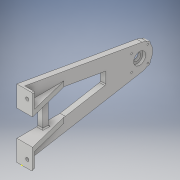
# Autodesk Inventor part: halter_seite
Saved by Autodesk Inventor 2017 (Build 210142000, 142)
## iProperties
Part Number: halter_seite
Material: Generisch
Document SubType Name: Modeling
Designer: Fabio
Density: 1 g/cm^3
Appearance: Vorgabe
Author: Fabio
Autodesk Inventor part; units mm, degrees
ref_plane "YZ Plane" through (0, 0, 0) normal (1, 0, 0) x (0, 1, 0)
ref_plane "XZ Plane" through (0, 0, 0) normal (0, 1, 0) x (-1, 0, 0)
ref_plane "XY Plane" through (0, 0, 0) normal (0, 0, 1) x (1, 0, 0)
sketch "Skizze1" plane through (0, 0, 0) normal (1, 0, 0) x (0, 1, 0)
  arc A0 (250, 65.0592) -> (229.3412, 89.6794) centre (225, 65.0592) ccw
  line L0 (225, 65.0592) -> (229.3412, 89.6794) construction
  line L1 (225, 65.0592) -> (250, 65.0592) construction
  line L2 (229.3412, 89.6794) -> (0, 130.1185)
  line L3 (0, 130.1185) -> (0, 90.1185)
  arc A1 (229.3412, 40.439) -> (250, 65.0592) centre (225, 65.0592) ccw
  line L4 (229.3412, 40.439) -> (0, 0)
  line L5 (0, 0) -> (92.864, 0) construction
  line L6 (0, 0) -> (0, 40)
  line L7 (160, 76.5205) -> (160, 53.598)
  line L8 (40, 90.1185) -> (40, 40)
  line L9 (50, 40) -> (50, 90.1185)
  line L10 (82.882, 90.1185) -> (160, 76.5205)
  line L11 (82.882, 40) -> (160, 53.598)
  line L12 (0, 40) -> (40, 40)
  line L13 (50, 40) -> (82.882, 40)
  line L14 (0, 90.1185) -> (40, 90.1185)
  line L15 (50, 90.1185) -> (82.882, 90.1185)
  dimension "d21" = 80
  dimension "d24" = 25
  dimension "d68" = 250
  dimension "d73" = 80
  dimension "d88" = 130.1185
  dimension "d91" = 10
  dimension "d92" = 25
  dimension "d93" = 25
  dimension "d94" = 40
  dimension "d127" = 110
  dimension "d160" = 40
  dimension "d161" = 40
  dimension "d162" = 80
  dimension "d163" = 32.882
  dimension "d164" = 32.882
  constraints: 32 end point, 5 horizontal, 4 point on circle, 4 vertical, 2 centre point, 2 symmetric about line, 1 coincident, 1 parallel, 1 other
  measures "d21" angle of L1 L0
  measures "d24" radius of A0
  measures "d68" distance from line of L1.end L3
  measures "d73" angle of L3 L2
  measures "d88" distance of point (0, 0) L2.end
  measures "d91" distance between parallel lines of L8 L9
  measures "d92" distance between parallel lines of L2 L10
  measures "d93" distance between parallel lines of L4 L11
  measures "d94" distance from line of L8 L3.end
  measures "d127" distance between parallel lines of L9 L7
  measures "d160" distance of L2.end L3.end
  measures "d161" distance of L4.end L6.end
  measures "d162" angle of L4 L6
  measures "d163" distance of L9.end L10.start
  measures "d164" distance of L9.start L11.start
extrude "Extrusion2" add sketch "Skizze1" along normal blind 10
sketch "Skizze7" plane through (10, 0, 0) normal (1, 0, 0) x (0, 0, -1)
  arc A0 (-40.439, 229.3412) -> (-89.6794, 229.3412) centre (-65.0592, 225) ccw projected
  point P0 (0, 0)
  constraints: 1 coincident
hole "Bohrung6" at (10, 225, 65.0592) direction (-1, 0, 0) diameter 14 end through all
fillet "Rundung1" radius 2 5 edges at (5, 160, 76.5205) (5, 40, 90.1185) (5, 50, 40) (5, 160, 53.598) (5, 40, 40)
sketch "Skizze13" plane through (0, 0, 0) normal (-1, 0, 0) x (0, 0, 1)
  line L0 (80.5592, 240.5) -> (80.5592, 209.5)
  line L1 (80.5592, 209.5) -> (49.5592, 209.5)
  line L2 (49.5592, 209.5) -> (49.5592, 240.5)
  line L3 (49.5592, 240.5) -> (80.5592, 240.5)
  line L4 (80.5592, 240.5) -> (49.5592, 209.5) construction
  line L5 (80.5592, 209.5) -> (49.5592, 240.5) construction
  line L6 (80.5592, 240.5) -> (111.5592, 240.5) construction
  point P0 (0, 0)
  point P1 (65.0592, 225)
  dimension "d145" = 31
  dimension "d146" = 90
  dimension "d147" = 31
  constraints: 14 end point, 4 coincident, 2 midpoint, 2 parallel, 2 perpendicular, 1 horizontal
  measures "d145" distance of L0.start L0.end
  measures "d146" angle of L0 L6
  measures "d147" distance of L0.end L1.end
hole "Bohrung10" at (0, 209.5, 80.5592) at (0, 240.5, 80.5592) at (0, 240.5, 49.5592) at (0, 209.5, 49.5592) direction (1, 0, 0) diameter 3 end through all counterbore diameter 5 counterbore depth 5
sketch "Skizze14" plane through (10, 0, 0) normal (1, 0, 0) x (0, 0, -1)
  line L0 (-90.1185, 0) -> (-90.1185, 38) projected
  line L1 (-90.1185, 0) -> (-100.1185, 0)
  line L2 (-100.1185, 0) -> (-100.1185, 80)
  line L3 (-100.1185, 80) -> (-90.1185, 80)
  line L4 (-90.1185, 80) -> (-90.1185, 0)
  line L5 (-40, 0) -> (0, 0) projected
  line L6 (-40, 0) -> (-30, 0)
  line L7 (-30, 0) -> (-30, 80)
  line L8 (-30, 80) -> (-40, 80)
  line L9 (-40, 80) -> (-40, 0)
  dimension "d165" = 10
  dimension "d166" = 80
  dimension "d167" = 10
  dimension "d168" = 80
  constraints: 16 end point, 4 parallel, 2 horizontal, 2 perpendicular
  measures "d165" distance of L2.end L3.end
  measures "d166" distance of L1.end L2.end
  measures "d167" distance of L8.end L7.end
  measures "d168" distance of L7.end L6.end
sketch "Skizze15" plane through (10, 0, 0) normal (1, 0, 0) x (0, 0, -1)
  circle A0 centre (-65.0592, 225) radius 7 projected
  circle A1 centre (-65.0592, 225) radius 11.5
  point P0 (0, 0)
  dimension "d157" = 23
  constraints: 1 centre point, 1 coincident
  measures "d157" diameter of A1
extrude "Extrusion4" cut sketch "Skizze15" against normal blind 5
sketch "Skizze16" plane through (10, 0, 0) normal (1, 0, 0) x (0, 0, -1)
  point P0 (0, 0)
sketch "Skizze17" plane through (10, 0, 0) normal (1, 0, 0) x (0, 0, -1)
  point P0 (0, 0)
extrude "Extrusion5" add sketch "Skizze14" along normal blind 20
sketch "Skizze18" plane through (10, 0, 100.1185) normal (0, 0, 1) x (1, 0, 0)
  line L0 (0, 0) -> (0, 80) projected
  line L1 (0, 0) -> (20, 0) projected
  line L2 (20, 80) -> (20, 0) projected
  line L3 (0, 80) -> (20, 80) projected
  line L4 (20, 80) -> (20, 0) projected
  line L5 (20, 0) -> (0, 80)
  line L6 (20, 80) -> (0, 80)
  point P0 (-10, 0)
  constraints: 4 end point, 1 collinear
sketch "Skizze19" plane through (10, 0, 0) normal (1, 0, 0) x (0, 0, -1)
  line L0 (0, 0) -> (-40.439, 229.3412) projected
  arc A0 (-40.439, 229.3412) -> (-89.6794, 229.3412) centre (-65.0592, 225) ccw projected
  line L1 (-89.6794, 229.3412) -> (-130.1185, 0) projected
  line L2 (-130.1185, 0) -> (-100.1185, 0) projected
  line L3 (-100.1185, 0) -> (-100.1185, 80) projected
  line L4 (-90.1185, 80) -> (-90.1185, 82.882) projected
  line L5 (-90.1185, 82.882) -> (-76.8119, 158.3473) projected
  arc A1 (-74.8423, 160) -> (-76.8119, 158.3473) centre (-74.8423, 158) ccw projected
  line L6 (-74.8423, 160) -> (-55.2762, 160) projected
  arc A2 (-53.3066, 158.3473) -> (-55.2762, 160) centre (-55.2762, 158) ccw projected
  line L7 (-53.3066, 158.3473) -> (-40, 82.882) projected
  line L8 (-40, 82.882) -> (-40, 80) projected
  line L9 (-30, 80) -> (-30, 0) projected
  line L10 (-30, 0) -> (0, 0) projected
  circle A3 centre (-65.0592, 225) radius 11.5 projected
  circle A4 centre (-49.5592, 240.5) radius 1.5 projected
  circle A5 centre (-80.5592, 209.5) radius 1.5 projected
  circle A6 centre (-80.5592, 240.5) radius 1.5 projected
  circle A7 centre (-49.5592, 209.5) radius 1.5 projected
  line L11 (-90.1185, 80) -> (-90.1185, 0) projected
  line L12 (-105.1185, 80) -> (-90.1185, 80) projected
  line L13 (-105.1185, 0) -> (-105.1185, 80) projected
  line L14 (-105.1185, 0) -> (-90.1185, 0) projected
  line L15 (-130.1185, 0) -> (-105.1185, 0)
  line L16 (-100.1185, 0) -> (-100.1185, 80) projected
  line L17 (-100.1185, 0) -> (-100.1185, 5)
  line L18 (-100.1185, 0) -> (-95.1185, 0) construction
  line L19 (-100.1185, 5) -> (-129.2368, 5)
  line L20 (-130.1185, 0) -> (-129.2368, 5)
  line L21 (-100.1185, 80) -> (-90.1185, 80) projected
  line L22 (-40, 80) -> (-30, 80) projected
  dimension "d173" = 5
  dimension "d174" = 90
  constraints: 10 end point, 3 perpendicular, 1 horizontal, 1 point on line, 1 vertical, 1 other
  measures "d173" distance of L2.end L17.end
  measures "d174" angle of L18 L17
sketch "Skizze20" plane through (10, 0, 0) normal (1, 0, 0) x (0, 0, -1)
  point P0 (0, 0)
extrude "Extrusion7" add sketch "Skizze19" along normal blind 20 contours L19 L13 L2 L1 | L19 L3 L2 L13
sketch "Skizze21" plane through (10, 0, 0) normal (1, 0, 0) x (0, 0, -1)
  circle A0 centre (-49.5592, 209.5) radius 1.5 projected
  circle A1 centre (-80.5592, 240.5) radius 1.5 projected
  circle A2 centre (-80.5592, 209.5) radius 1.5 projected
  circle A3 centre (-49.5592, 240.5) radius 1.5 projected
  circle A4 centre (-65.0592, 225) radius 11.5 projected
  line L0 (-129.2368, 5) -> (-100.1185, 5) projected
  line L1 (-100.1185, 5) -> (-100.1185, 80) projected
  line L2 (-100.1185, 80) -> (-90.1185, 80) projected
  line L3 (-90.1185, 80) -> (-90.1185, 82.882) projected
  line L4 (-90.1185, 82.882) -> (-76.8119, 158.3473) projected
  arc A5 (-74.8423, 160) -> (-76.8119, 158.3473) centre (-74.8423, 158) ccw projected
  line L5 (-74.8423, 160) -> (-55.2762, 160) projected
  arc A6 (-53.3066, 158.3473) -> (-55.2762, 160) centre (-55.2762, 158) ccw projected
  line L6 (-53.3066, 158.3473) -> (-40, 82.882) projected
  line L7 (-40, 82.882) -> (-40, 80) projected
  line L8 (-40, 80) -> (-30, 80) projected
  line L9 (-30, 80) -> (-30, 0) projected
  line L10 (-30, 0) -> (0, 0) projected
  line L11 (0, 0) -> (-40.439, 229.3412) projected
  arc A7 (-40.439, 229.3412) -> (-89.6794, 229.3412) centre (-65.0592, 225) ccw projected
  line L12 (-89.6794, 229.3412) -> (-129.2368, 5) projected
  line L13 (-40, 0) -> (-30, 0) projected
  line L14 (-30, 0) -> (-30, 80) projected
  line L15 (-30, 80) -> (-40, 80) projected
  line L16 (-40, 80) -> (-40, 0) projected
  line L17 (0, 0) -> (-0.8816, 5)
  line L18 (-30, 80) -> (-30, 0) projected
  line L19 (-30, 5) -> (-30, 0)
  line L20 (-30, 0) -> (0, 0)
  line L21 (-30, 5) -> (-0.8816, 5)
  dimension "d177" = 5
  constraints: 8 end point, 2 point on line, 1 collinear, 1 perpendicular, 1 vertical
  measures "d177" distance between parallel lines of L10 L21
extrude "Extrusion8" add sketch "Skizze21" along normal blind 20 contours L11 L10 L9 L21
extrude "Extrusion9" cut sketch "Skizze18" along normal through all both and the other way through all contours L3 L2 L5
sketch "Skizze22" plane through (10, 5, 30) normal (0, 1, 0) x (1, 0, 0)
  line L0 (0, -60.1185) -> (20, -60.1185) construction
  line L1 (20, -100.1185) -> (20, -60.1185) construction
  line L2 (20, -10) -> (20, 30) construction
  line L3 (20, -10) -> (0, -10) construction
  point P0 (-10, 30)
  point P1 (10, -85.1185)
  point P2 (10, 15)
  dimension "d182" = 25
  dimension "d183" = 10
  dimension "d184" = 10
  dimension "d185" = 25
  measures "d182" distance from line of L0 point (10, -85.118)
  measures "d183" distance from line of L1 point (10, -85.118)
  measures "d184" distance from line of L2 point (10, 15)
  measures "d185" distance from line of point (10, 15) L3
hole "Bohrung11" at (20, 5, 115.1185) at (20, 5, 15) direction (0, -1, 0) diameter 6.3 end through all
fillet "Rundung2" radius 2 5 edges at (10, 44, 90.1185) (5, 50, 90.1185) (29.375, 2.5, 0.4408) (29.375, 2.5, 129.6777) (10, 45, 40)
sketch "Skizze23" plane through (0, 0, 0) normal (-1, 0, 0) x (0, 0, 1)
  circle A0 centre (80.5592, 240.5) radius 2.5 projected
  circle A1 centre (80.5592, 240.5) radius 5
  circle A2 centre (49.5592, 240.5) radius 2.5 projected
  circle A3 centre (49.5592, 240.5) radius 5
  arc A4 (89.6794, 229.3412) -> (40.439, 229.3412) centre (65.0592, 225) ccw projected
  point P0 (0, 0)
  dimension "d194" = 10
  dimension "d195" = 10
  constraints: 2 centre point, 2 coincident
  measures "d194" diameter of A1
  measures "d195" diameter of A3
extrude "Extrusion10" add sketch "Skizze23" against normal blind 10
